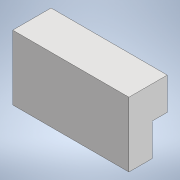
# Autodesk Inventor part: Part16
Saved by Autodesk Inventor 2022.3 (Build 263350000, 350)
## iProperties
Created: 2022-11-17
Part Number: Part16
Material: Generic
Document SubType Name: Modeling
Designer: komputer
Density: 1 g/cm^3
Appearance: Default
Author: komputer
Autodesk Inventor part; units mm, degrees
ref_plane "YZ Plane" through (0, 0, 0) normal (1, 0, 0) x (0, 1, 0)
ref_plane "XZ Plane" through (0, 0, 0) normal (0, 1, 0) x (-1, 0, 0)
ref_plane "XY Plane" through (0, 0, 0) normal (0, 0, 1) x (1, 0, 0)
sketch "Sketch1" plane through (0, 0, 0) normal (0, 0, 1) x (1, 0, 0)
  line L0 (25, -7) -> (50, -7) projected
  line L1 (50, 45.5218) -> (50, -7) projected
  line L2 (50, 45.5218) -> (11.4158, 45.5218) projected
  line L3 (11.4158, 45.5218) -> (11.4158, 48.5218) projected
  line L4 (11.4158, 48.5218) -> (-11.4158, 48.5218) projected
  line L5 (-11.4158, 48.5218) -> (-11.4158, 45.5218) projected
  line L6 (-11.4158, 45.5218) -> (-50, 45.5218) projected
  line L7 (-50, 45.5218) -> (-50, -7) projected
  line L8 (-50, -7) -> (-25, -7) projected
  line L9 (-25, -7) -> (-25, -24) projected
  line L10 (-25, -24) -> (-32.4371, -24) projected
  line L11 (-32.4371, -24) -> (-32.4371, -28) projected
  line L12 (-32.4371, -28) -> (-25, -28) projected
  line L13 (-25, -28) -> (-25, -35) projected
  line L14 (-25, -35) -> (25, -35) projected
  line L15 (25, -35) -> (25, -28) projected
  line L16 (25, -28) -> (30.7079, -28) projected
  line L17 (30.7079, -28) -> (30.7079, -24) projected
  line L18 (30.7079, -24) -> (25, -24) projected
  line L19 (25, -24) -> (25, -7) projected
  circle A0 centre (-11.4158, 26.1989) radius 1.6 projected
  circle A1 centre (20.9961, 37.6953) radius 1.6 projected
  circle A2 centre (-20.9961, 37.6953) radius 1.6 projected
  circle A3 centre (11.4158, 26.1989) radius 1.6 projected
  line L20 (15.6, -21.3595) -> (2, -21.3595) projected
  line L21 (-2, -21.3109) -> (-15.6, -21.3109) projected
  line L22 (-2.4, -19.4751) -> (-15.6, -19.4751)
  line L23 (2.4, -19.5236) -> (15.6, -19.5236)
  line L24 (50, -7) -> (-50, -7)
  line L25 (-50, -7) -> (-50, 20.7683)
  line L26 (-50, 20.7683) -> (50, 20.7683)
  line L27 (50, 20.7683) -> (50, -7)
  point P0 (0, 0)
  constraints: 12 end point, 3 horizontal, 2 parallel, 1 perpendicular, 1 point on line, 4 other
extrude "Extrusion1" add sketch "Sketch1" along normal blind 13 contours L24 L8 L7 L26 L1 L0
sketch "Sketch2" plane through (0, 0, 13) normal (0, 0, 1) x (1, 0, 0)
  line L0 (25, -7) -> (50, -7) projected
  line L1 (50, 45.5218) -> (50, -7) projected
  line L2 (50, 45.5218) -> (11.4158, 45.5218) projected
  line L3 (11.4158, 45.5218) -> (11.4158, 48.5218) projected
  line L4 (11.4158, 48.5218) -> (-11.4158, 48.5218) projected
  line L5 (-11.4158, 48.5218) -> (-11.4158, 45.5218) projected
  line L6 (-11.4158, 45.5218) -> (-50, 45.5218) projected
  line L7 (-50, 45.5218) -> (-50, -7) projected
  line L8 (-50, -7) -> (-25, -7) projected
  line L9 (-25, -7) -> (-25, -24) projected
  line L10 (-25, -24) -> (-32.4371, -24) projected
  line L11 (-32.4371, -24) -> (-32.4371, -28) projected
  line L12 (-32.4371, -28) -> (-25, -28) projected
  line L13 (-25, -28) -> (-25, -35) projected
  line L14 (-25, -35) -> (25, -35) projected
  line L15 (25, -35) -> (25, -28) projected
  line L16 (25, -28) -> (30.7079, -28) projected
  line L17 (30.7079, -28) -> (30.7079, -24) projected
  line L18 (30.7079, -24) -> (25, -24) projected
  line L19 (25, -24) -> (25, -7) projected
  circle A0 centre (-11.4158, 26.1989) radius 1.6 projected
  circle A1 centre (20.9961, 37.6953) radius 1.6 projected
  circle A2 centre (-20.9961, 37.6953) radius 1.6 projected
  circle A3 centre (11.4158, 26.1989) radius 1.6 projected
  line L20 (50, 20.7683) -> (-50, 20.7683) projected
  line L21 (-50, 20.7683) -> (50, 20.7683)
  line L22 (50, 20.7683) -> (50, -35)
  line L23 (50, -35) -> (-50, -35)
  line L24 (-50, -35) -> (-50, 20.7683)
  point P0 (0, 0)
  constraints: 8 end point, 2 parallel, 1 horizontal, 1 perpendicular
extrude "Extrusion2" add sketch "Sketch2" along normal blind 20 contours L19 L18 L17 L16 L15 L14 L13 L12 L11 L10 L9 L8 L7 L20 L1 L0 | L0 L22 L23 L15 L16 L17 L18 L19 | L8 L9 L10 L11 L12 L13 L23 L24
body "Solid1"
